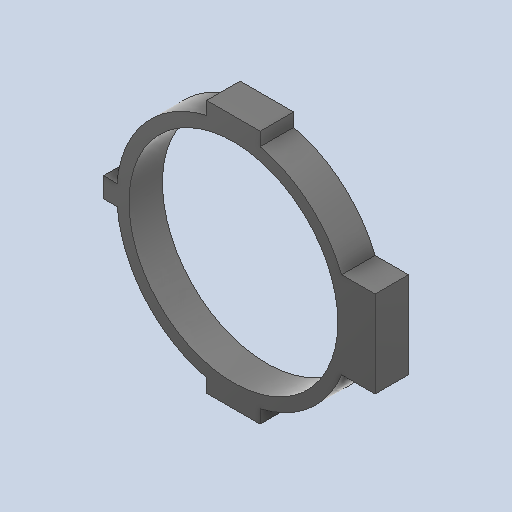
# Autodesk Inventor part: celestronTubeBracket
Saved by Autodesk Inventor 2022 (Build 260153070, 153G)
## iProperties
Created: 2020-07-21
Part Number: celestronTubeBracket
Material: Aluminum 6061
Document SubType Name: Modeling
Designer: robst
Density: 2.7 g/cm^3
Appearance: Smooth - Black
Mass: 501.045 g
Surface Area: 442.424 cm^2
Volume: 185.572 cm^3
Author: robst
Autodesk Inventor part; units mm, degrees
ref_plane "YZ Plane" through (0, 0, 0) normal (1, 0, 0) x (0, 1, 0)
ref_plane "XZ Plane" through (0, 0, 0) normal (0, 1, 0) x (-1, 0, 0)
ref_plane "XY Plane" through (0, 0, 0) normal (0, 0, 1) x (1, 0, 0)
sketch "Sketch1" plane through (0, 0, 0) normal (0, 0, 1) x (1, 0, 0)
  circle A0 centre (0, 0) radius 79.375
  line L0 (82.2618, 32.9086) -> (107.6618, 32.9086)
  line L1 (107.6618, 32.9086) -> (107.6618, -0.1114)
  line L2 (-88.5728, 7.62) -> (-98.7328, 7.62)
  line L3 (-98.7328, 7.62) -> (-98.7328, 0)
  line L4 (0, 96.3985) -> (20.32, 96.3985)
  line L5 (20.32, 96.3985) -> (20.32, 86.2385)
  line L6 (82.2618, -32.9086) -> (107.6618, -32.9086)
  line L7 (107.6618, -32.9086) -> (107.6618, -0.1114)
  line L8 (-88.2741, -7.5943) -> (-98.7328, -7.5943)
  line L9 (-98.7328, -7.5943) -> (-98.7328, 0)
  line L10 (0, 96.3985) -> (-20.32, 96.3985)
  line L11 (-20.32, 96.3985) -> (-20.32, 86.5466)
  arc A1 (-88.2741, -7.5943) -> (-20.32, -86.2385) centre (0, 0) ccw
  arc A2 (-20.32, 86.5466) -> (-88.5728, 7.62) centre (0, 0) ccw
  arc A3 (20.32, -86.2385) -> (82.2618, -32.9086) centre (0, 0) ccw
  arc A4 (82.2618, 32.9086) -> (20.32, 86.2385) centre (0, 0) ccw
  line L12 (-88.9, 0) -> (88.9, 0) construction
  line L13 (0, -96.3985) -> (20.32, -96.3985)
  line L14 (20.32, -96.3985) -> (20.32, -86.2385)
  line L15 (0, -96.3985) -> (-20.32, -96.3985)
  line L16 (-20.32, -96.3985) -> (-20.32, -86.2385)
  arc A5 (-20.32, 86.5466) -> (-88.5728, 7.62) centre (0, 0) ccw
  arc A6 (82.2618, 32.9086) -> (20.32, 86.2385) centre (0, 0) ccw
  arc A7 (-88.2741, -7.5943) -> (-20.32, -86.2385) centre (0, 0) ccw
  arc A8 (20.32, -86.2385) -> (82.2618, -32.9086) centre (0, 0) ccw
  line L17 (0, 0) -> (0, 96.3985) construction
  line L18 (0, 0) -> (0, -96.3985) construction
  dimension "d2" = 25.4
  dimension "d5" = 10.16
  dimension "d7" = 10.16
  dimension "d8" = 7.62
  dimension "d10" = 33.02
  dimension "d14" = 158.75
  dimension "d15" = 177.8
  dimension "d24" = 20.32
  dimension "d25" = 20.32
  dimension "d26" = 40.64
  constraints: 38 end point, 16 point on circle, 9 centre point, 4 horizontal, 3 coincident, 3 perpendicular, 3 symmetric about line, 2 vertical
  measures "d2" distance of L0.start L0.end
  measures "d5" distance of L4.end L5.end
  measures "d7" distance of L2.start L2.end
  measures "d8" distance of L2.end L3.end
  measures "d10" distance of L0.end L1.end
  measures "d14" diameter of A0
  measures "d15" diameter of A2
  measures "d24" distance between parallel lines of L5 L17
  measures "d25" distance between parallel lines of L11 L17
  measures "d26" distance between parallel lines of L14 L16
extrude "Extrusion2" add sketch "Sketch1" along normal mid plane 25.4
body "Solid2"
